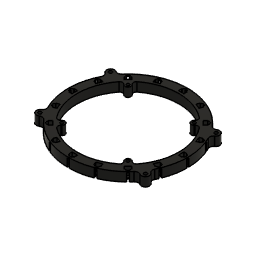
ir_ring_v1 (Autodesk Fusion 360 design; units mm, degrees)
Autodesk Fusion 360 part; units mm, degrees
note: some values were not read from the file. Set by a fixed rule: which sketch regions a step uses.
(part 1 of 2)
sketch "Sketch1" plane through (0, 0, 0) normal (0, 1, 0) x (1, 0, 0)
  circle A0 centre (0, 0) radius 105
  line L0 (0, 0) -> (74.2462, 74.2462) construction
  line L1 (0, 0) -> (105, 0) construction
  line L2 (74.2462, 74.2462) -> (56.5685, 91.9239) construction
  line L3 (56.5685, 91.9239) -> (54.4334, 89.7887) construction
  line L4 (54.4334, 89.7887) -> (43.8268, 79.1821)
  line L5 (43.8268, 79.1821) -> (61.5044, 61.5044)
  line L6 (89.7887, 54.4334) -> (79.1821, 43.8268)
  line L7 (79.1821, 43.8268) -> (61.5044, 61.5044)
  line L8 (-54.4334, 89.7887) -> (-43.8268, 79.1821)
  line L9 (-43.8268, 79.1821) -> (-61.5044, 61.5044)
  line L10 (-79.1821, 43.8268) -> (-61.5044, 61.5044)
  line L11 (-89.7887, 54.4334) -> (-79.1821, 43.8268)
  line L12 (-89.7887, -54.4334) -> (-79.1821, -43.8268)
  line L13 (-79.1821, -43.8268) -> (-61.5044, -61.5044)
  line L14 (-43.8268, -79.1821) -> (-61.5044, -61.5044)
  line L15 (-54.4334, -89.7887) -> (-43.8268, -79.1821)
  line L16 (54.4334, -89.7887) -> (43.8268, -79.1821)
  line L17 (43.8268, -79.1821) -> (61.5044, -61.5044)
  line L18 (79.1821, -43.8268) -> (61.5044, -61.5044)
  line L19 (89.7887, -54.4334) -> (79.1821, -43.8268)
  line L20 (61.5044, 61.5044) -> (58.5876, 58.5876) construction
  line L21 (58.5876, 58.5876) -> (47.3623, 69.8129) construction
  circle A1 centre (47.3623, 69.8129) radius 1.65
  circle A2 centre (69.8129, 47.3623) radius 1.65
  circle A3 centre (-47.3623, 69.8129) radius 1.65
  circle A4 centre (-69.8129, 47.3623) radius 1.65
  circle A5 centre (-69.8129, -47.3623) radius 1.65
  circle A6 centre (-47.3623, -69.8129) radius 1.65
  circle A7 centre (47.3623, -69.8129) radius 1.65
  circle A8 centre (69.8129, -47.3623) radius 1.65
  line L22 (0, 0) -> (0, 105) construction
  line L23 (0, 105) -> (45, 105) construction
  line L24 (45, 105) -> (45, 94.8683) construction
  line L25 (45, 94.8683) -> (0, 94.8683) construction
  line L26 (0, 94.8683) -> (0, 69.8683) construction
  line L27 (0, 69.8683) -> (0, 107.8683) construction
  circle A9 centre (0, 107.8683) radius 38
  line L28 (45, 94.8683) -> (23.4509, 77.9676)
  line L29 (-45, 94.8683) -> (-23.4509, 77.9676)
  circle A10 centre (0, 0) radius 61
  line L30 (0, 0) -> (11.9005, 59.8279) construction
  line L31 (7.9774, 60.6083) -> (6.8068, 54.7236)
  arc A11 (6.8068, 54.7236) -> (14.6531, 53.1628) centre (10.73, 53.9432) ccw
  line L32 (14.6531, 53.1628) -> (15.8237, 59.0475)
  arc A12 (15.8237, 59.0475) -> (7.9774, 60.6083) centre (11.9005, 59.8279) ccw
  line L33 (11.9005, 59.8279) -> (10.73, 53.9432) construction
  circle A13 centre (10.73, 53.9432) radius 1.65
  line L34 (-60.6083, 7.9774) -> (-54.7236, 6.8068)
  line L35 (-53.1628, 14.6531) -> (-59.0475, 15.8237)
  arc A14 (-54.7236, 6.8068) -> (-53.1628, 14.6531) centre (-53.9432, 10.73) ccw
  circle A15 centre (-53.9432, 10.73) radius 1.65
  line L36 (-7.9774, -60.6083) -> (-6.8068, -54.7236)
  line L37 (-14.6531, -53.1628) -> (-15.8237, -59.0475)
  arc A16 (-6.8068, -54.7236) -> (-14.6531, -53.1628) centre (-10.73, -53.9432) ccw
  circle A17 centre (-10.73, -53.9432) radius 1.65
  line L38 (60.6083, -7.9774) -> (54.7236, -6.8068)
  line L39 (53.1628, -14.6531) -> (59.0475, -15.8237)
  arc A18 (54.7236, -6.8068) -> (53.1628, -14.6531) centre (53.9432, -10.73) ccw
  circle A19 centre (53.9432, -10.73) radius 1.65
  dimension "d1" = 210
  dimension "d2" = 45
  dimension "d3" = 25
  dimension "d4" = 15
  dimension "d6" = 360
  dimension "d7" = 4.125
  dimension "d8" = 15.875
  dimension "d9" = 3.3
  dimension "d11" = 360
  dimension "d12" = 45
  dimension "d13" = 25
  dimension "d14" = 38
  dimension "d35" = 122
  dimension "d36" = 11.25
  dimension "d37" = 6
  dimension "d38" = 8
  dimension "d39" = 3.3
  dimension "d41" = 360
  constraint coincident A0.centre L0.start
  constraint horizontal L1
  constraint coincident A0 L0.end
  constraint tangent A0 L2
  constraint coincident A0 L3.end
  constraint perpendicular L2 L3
  constraint perpendicular L2 L4
  constraint coincident L0 L5.end
  constraint perpendicular L0 L5
  constraint symmetric L0 L3.end L6.start
  constraint symmetric L0 L4.end L6.end
  constraint symmetric L0 L5.end L7.end
  constraint perpendicular L7 L20
  constraint perpendicular L20 L21
  constraint coincident L21.end A1.centre
  constraint symmetric L0 A1 A2
  constraint coincident A0 L22.end
  constraint perpendicular L1 L22
  constraint perpendicular L22 L23
  constraint coincident A0 L24.end
  constraint perpendicular L23 L24
  constraint coincident L22 L25.end
  constraint perpendicular L22 L25
  constraint perpendicular L25 L26
  constraint parallel L22 L27
  constraint coincident L27.end A9.centre
  constraint coincident L26.end A9
  constraint coincident A9 L28.end
  constraint tangent A9 L28
  constraint symmetric L22 L24.end L29.start
  constraint symmetric L22 L28.end L29.end
  constraint coincident A10 L30.end
  constraint tangent L31 A11
  constraint tangent A11 L32
  constraint parallel L31 L32
  constraint tangent L32 A12
  constraint tangent L31 A12
  constraint coincident L30 A11.centre
  constraint parallel L30 L33
  constraint coincident L30.end A12.centre
  constraint concentric A11 A13
  measures "d1" diameter of A0
  measures "d2" angle of L0 L1
  measures "d3" distance of L0.end L2.end
  measures "d4" distance of L3.end L4.end
  measures "d7" distance of L5.end L20.end
  measures "d8" distance of L20.end L21.end
  measures "d9" diameter of A1
  measures "d12" distance of L22.end L23.end
  measures "d13" distance of L25.end L26.end
  measures "d14" distance of L26.end L27.end
  measures "d35" diameter of A10
  measures "d36" angle of L22 L30
  measures "d37" distance of L30.end A11.centre
  measures "d38" diameter of A11
  measures "d39" diameter of A13
sketch "Sketch2" plane through (0, 38, 0) normal (0, 1, 0) x (-1, 0, 0)
  circle A0 centre (-69.8129, -47.3623) radius 1.65
  circle A1 centre (-47.3623, -69.8129) radius 1.65
  arc A2 (-50.2791, -72.7297) -> (-44.4455, -66.8961) centre (-47.3623, -69.8129) ccw
  line L0 (-44.4455, -66.8961) -> (-66.8961, -44.4455)
  arc A3 (-66.8961, -44.4455) -> (-72.7297, -50.2791) centre (-69.8129, -47.3623) ccw
  line L1 (-72.7297, -50.2791) -> (-50.2791, -72.7297)
  circle A4 centre (-47.3623, -69.8129) radius 1.65
  circle A5 centre (-69.8129, 47.3623) radius 1.65
  circle A6 centre (-47.3623, 69.8129) radius 1.65
  circle A7 centre (47.3623, 69.8129) radius 1.65
  circle A8 centre (69.8129, 47.3623) radius 1.65
  circle A9 centre (69.8129, -47.3623) radius 1.65
  circle A10 centre (47.3623, -69.8129) radius 1.65
  circle A11 centre (-69.8129, -47.3623) radius 1.65
  line L2 (54.4334, -89.7887) -> (43.8268, -79.1821)
  line L3 (43.8268, -79.1821) -> (79.1821, -43.8268)
  line L4 (79.1821, -43.8268) -> (89.7887, -54.4334)
  arc A12 (89.7887, -54.4334) -> (89.7887, 54.4334) centre (0, 0) ccw
  line L5 (89.7887, 54.4334) -> (79.1821, 43.8268)
  line L6 (79.1821, 43.8268) -> (43.8268, 79.1821)
  line L7 (43.8268, 79.1821) -> (54.4334, 89.7887)
  arc A13 (54.4334, 89.7887) -> (-54.4334, 89.7887) centre (0, 0) ccw
  line L8 (-54.4334, 89.7887) -> (-43.8268, 79.1821)
  line L9 (-43.8268, 79.1821) -> (-79.1821, 43.8268)
  line L10 (-79.1821, 43.8268) -> (-89.7887, 54.4334)
  arc A14 (-89.7887, 54.4334) -> (-89.7887, -54.4334) centre (0, 0) ccw
  line L11 (-89.7887, -54.4334) -> (-79.1821, -43.8268)
  line L12 (-79.1821, -43.8268) -> (-43.8268, -79.1821)
  line L13 (-43.8268, -79.1821) -> (-54.4334, -89.7887)
  arc A15 (-54.4334, -89.7887) -> (-45, -94.8683) centre (0, 0) ccw
  line L14 (-45, -94.8683) -> (-23.4509, -77.9676)
  arc A16 (23.4509, -77.9676) -> (-23.4509, -77.9676) centre (0, -107.8683) ccw
  line L15 (23.4509, -77.9676) -> (45, -94.8683)
  arc A17 (45, -94.8683) -> (54.4334, -89.7887) centre (0, 0) ccw
  line L16 (-79.1821, -43.8268) -> (-82.7176, -40.2912)
  line L17 (-43.8268, -79.1821) -> (-40.2912, -82.7176)
  line L18 (-40.2912, -82.7176) -> (-49.938, -92.3645)
  line L19 (-82.7176, -40.2912) -> (-92.3645, -49.938)
  line L20 (43.8268, -79.1821) -> (40.2912, -82.7176)
  line L21 (40.2912, -82.7176) -> (49.938, -92.3645)
  line L22 (82.7176, -40.2912) -> (92.3645, -49.938)
  line L23 (79.1821, -43.8268) -> (82.7176, -40.2912)
  line L24 (79.1821, 43.8268) -> (82.7176, 40.2912)
  line L25 (82.7176, 40.2912) -> (92.3645, 49.938)
  line L26 (40.2912, 82.7176) -> (49.938, 92.3645)
  line L27 (43.8268, 79.1821) -> (40.2912, 82.7176)
  line L28 (-43.8268, 79.1821) -> (-40.2912, 82.7176)
  line L29 (-40.2912, 82.7176) -> (-49.938, 92.3645)
  line L30 (-82.7176, 40.2912) -> (-92.3645, 49.938)
  line L31 (-79.1821, 43.8268) -> (-82.7176, 40.2912)
  circle A18 centre (-25.9723, -48.5997) radius 1.65
  circle A19 centre (-48.5997, -25.9723) radius 1.65
  circle A20 centre (25.9723, -48.5997) radius 1.65
  circle A21 centre (48.5997, -25.9723) radius 1.65
  circle A22 centre (25.9723, 48.5997) radius 1.65
  circle A23 centre (48.5997, 25.9723) radius 1.65
  circle A24 centre (-25.9723, 48.5997) radius 1.65
  circle A25 centre (-48.5997, 25.9723) radius 1.65
  circle A26 centre (-53.9432, 10.73) radius 1.65
  circle A27 centre (10.73, 53.9432) radius 1.65
  circle A28 centre (53.9432, -10.73) radius 1.65
  circle A29 centre (-10.73, -53.9432) radius 1.65
  arc A30 (-60.4795, 7.9518) -> (-15.798, -58.9188) centre (0, 0) ccw
  line L32 (-60.4795, 7.9518) -> (-54.7236, 6.8068)
  arc A31 (-54.7236, 6.8068) -> (-53.1628, 14.6531) centre (-53.9432, 10.73) ccw
  line L33 (-53.1628, 14.6531) -> (-58.9188, 15.798)
  arc A32 (7.9518, 60.4795) -> (-58.9188, 15.798) centre (0, 0) ccw
  line L34 (7.9518, 60.4795) -> (6.8068, 54.7236)
  arc A33 (6.8068, 54.7236) -> (14.6531, 53.1628) centre (10.73, 53.9432) ccw
  line L35 (14.6531, 53.1628) -> (15.798, 58.9188)
  arc A34 (60.4795, -7.9518) -> (15.798, 58.9188) centre (0, 0) ccw
  line L36 (60.4795, -7.9518) -> (54.7236, -6.8068)
  arc A35 (54.7236, -6.8068) -> (53.1628, -14.6531) centre (53.9432, -10.73) ccw
  line L37 (53.1628, -14.6531) -> (58.9188, -15.798)
  arc A36 (-7.9518, -60.4795) -> (58.9188, -15.798) centre (0, 0) ccw
  line L38 (-7.9518, -60.4795) -> (-6.8068, -54.7236)
  arc A37 (-6.8068, -54.7236) -> (-14.6531, -53.1628) centre (-10.73, -53.9432) ccw
  line L39 (-14.6531, -53.1628) -> (-15.798, -58.9188)
  dimension "d29" = 5
  dimension "d30" = 5
  dimension "d32" = 360
  constraint coincident L11.end L12.start
  constraint perpendicular L11 L16
  constraint coincident L12.end L13.start
  constraint perpendicular L13 L17
  constraint coincident A14 L19.end
  constraint perpendicular L16 L19
  constraint parallel L13 L18
  constraint coincident A15 L18.end
  measures "d29" distance of L11.end L16.end
  measures "d30" distance of L12.end L17.end
sketch "Sketch3" plane through (0, 0, 0) normal (0, -1, 0) x (1, 0, 0)
  circle A0 centre (47.3623, -69.8129) radius 1.65
  circle A1 centre (53.9432, 10.73) radius 1.65
  circle A2 centre (-10.73, 53.9432) radius 1.65
  circle A3 centre (-53.9432, -10.73) radius 1.65
  circle A4 centre (69.8129, -47.3623) radius 1.65
  circle A5 centre (10.73, -53.9432) radius 1.65
  circle A6 centre (69.8129, 47.3623) radius 1.65
  circle A7 centre (47.3623, 69.8129) radius 1.65
  circle A8 centre (-47.3623, 69.8129) radius 1.65
  circle A9 centre (-69.8129, 47.3623) radius 1.65
  circle A10 centre (-69.8129, -47.3623) radius 1.65
  circle A11 centre (-47.3623, -69.8129) radius 1.65
  arc A12 (15.3738, -56.786) -> (17.923, -58.3075) centre (17.3354, -56.3958) ccw
  line L0 (15.3738, -56.786) -> (14.6531, -53.1628)
  arc A13 (14.6531, -53.1628) -> (6.8068, -54.7236) centre (10.73, -53.9432) ccw
  line L1 (6.8068, -54.7236) -> (7.5275, -58.3467)
  arc A14 (5.7546, -60.728) -> (7.5275, -58.3467) centre (5.5659, -58.7369) ccw
  arc A15 (-58.3075, -17.923) -> (5.7546, -60.728) centre (0, 0) ccw
  arc A16 (-56.786, -15.3738) -> (-58.3075, -17.923) centre (-56.3958, -17.3354) ccw
  line L2 (-56.786, -15.3738) -> (-53.1628, -14.6531)
  arc A17 (-53.1628, -14.6531) -> (-54.7236, -6.8068) centre (-53.9432, -10.73) ccw
  line L3 (-54.7236, -6.8068) -> (-58.3467, -7.5275)
  arc A18 (-60.728, -5.7546) -> (-58.3467, -7.5275) centre (-58.7369, -5.5659) ccw
  arc A19 (-17.923, 58.3075) -> (-60.728, -5.7546) centre (0, 0) ccw
  arc A20 (-15.3738, 56.786) -> (-17.923, 58.3075) centre (-17.3354, 56.3958) ccw
  line L4 (-15.3738, 56.786) -> (-14.6531, 53.1628)
  arc A21 (-14.6531, 53.1628) -> (-6.8068, 54.7236) centre (-10.73, 53.9432) ccw
  line L5 (-6.8068, 54.7236) -> (-7.5275, 58.3467)
  arc A22 (-5.7546, 60.728) -> (-7.5275, 58.3467) centre (-5.5659, 58.7369) ccw
  arc A23 (58.3075, 17.923) -> (-5.7546, 60.728) centre (0, 0) ccw
  arc A24 (56.786, 15.3738) -> (58.3075, 17.923) centre (56.3958, 17.3354) ccw
  line L6 (56.786, 15.3738) -> (53.1628, 14.6531)
  arc A25 (53.1628, 14.6531) -> (54.7236, 6.8068) centre (53.9432, 10.73) ccw
  line L7 (54.7236, 6.8068) -> (58.3467, 7.5275)
  arc A26 (60.728, 5.7546) -> (58.3467, 7.5275) centre (58.7369, 5.5659) ccw
  arc A27 (17.923, -58.3075) -> (60.728, 5.7546) centre (0, 0) ccw
  arc A28 (-46.1329, -94.3226) -> (-44.02, -94.0997) centre (-45.2542, -92.526) ccw
  line L8 (-44.02, -94.0997) -> (-23.4509, -77.9676)
  arc A29 (23.4509, -77.9676) -> (-23.4509, -77.9676) centre (0, -107.8683) ccw
  line L9 (23.4509, -77.9676) -> (44.02, -94.0997)
  arc A30 (44.02, -94.0997) -> (46.1329, -94.3226) centre (45.2542, -92.526) ccw
  arc A31 (46.1329, -94.3226) -> (52.1873, -91.1125) centre (0, 0) ccw
  arc A32 (52.1873, -91.1125) -> (52.6075, -87.9628) centre (51.1933, -89.377) ccw
  line L10 (52.6075, -87.9628) -> (45.241, -80.5963)
  arc A33 (45.241, -77.7679) -> (45.241, -80.5963) centre (46.6552, -79.1821) ccw
  line L11 (45.241, -77.7679) -> (77.7679, -45.241)
  arc A34 (80.5963, -45.241) -> (77.7679, -45.241) centre (79.1821, -46.6552) ccw
  line L12 (80.5963, -45.241) -> (87.9628, -52.6075)
  arc A35 (87.9628, -52.6075) -> (91.1125, -52.1873) centre (89.377, -51.1933) ccw
  arc A36 (91.1125, -52.1873) -> (91.1125, 52.1873) centre (0, 0) ccw
  arc A37 (91.1125, 52.1873) -> (87.9628, 52.6075) centre (89.377, 51.1933) ccw
  line L13 (87.9628, 52.6075) -> (80.5963, 45.241)
  arc A38 (77.7679, 45.241) -> (80.5963, 45.241) centre (79.1821, 46.6552) ccw
  line L14 (77.7679, 45.241) -> (45.241, 77.7679)
  arc A39 (45.241, 80.5963) -> (45.241, 77.7679) centre (46.6552, 79.1821) ccw
  line L15 (45.241, 80.5963) -> (52.6075, 87.9628)
  arc A40 (52.6075, 87.9628) -> (52.1873, 91.1125) centre (51.1933, 89.377) ccw
  arc A41 (52.1873, 91.1125) -> (-52.1873, 91.1125) centre (0, 0) ccw
  arc A42 (-52.1873, 91.1125) -> (-52.6075, 87.9628) centre (-51.1933, 89.377) ccw
  line L16 (-52.6075, 87.9628) -> (-45.241, 80.5963)
  arc A43 (-45.241, 77.7679) -> (-45.241, 80.5963) centre (-46.6552, 79.1821) ccw
  line L17 (-45.241, 77.7679) -> (-77.7679, 45.241)
  arc A44 (-80.5963, 45.241) -> (-77.7679, 45.241) centre (-79.1821, 46.6552) ccw
  line L18 (-80.5963, 45.241) -> (-87.9628, 52.6075)
  arc A45 (-87.9628, 52.6075) -> (-91.1125, 52.1873) centre (-89.377, 51.1933) ccw
  arc A46 (-91.1125, 52.1873) -> (-91.1125, -52.1873) centre (0, 0) ccw
  arc A47 (-91.1125, -52.1873) -> (-87.9628, -52.6075) centre (-89.377, -51.1933) ccw
  line L19 (-87.9628, -52.6075) -> (-80.5963, -45.241)
  arc A48 (-77.7679, -45.241) -> (-80.5963, -45.241) centre (-79.1821, -46.6552) ccw
  line L20 (-77.7679, -45.241) -> (-45.241, -77.7679)
  arc A49 (-45.241, -80.5963) -> (-45.241, -77.7679) centre (-46.6552, -79.1821) ccw
  line L21 (-45.241, -80.5963) -> (-52.6075, -87.9628)
  arc A50 (-52.6075, -87.9628) -> (-52.1873, -91.1125) centre (-51.1933, -89.377) ccw
  arc A51 (-52.1873, -91.1125) -> (-46.1329, -94.3226) centre (0, 0) ccw
  circle A52 centre (0, 0) radius 60
  circle A53 centre (0, 0) radius 40
  dimension "d46" = 120
  dimension "d47" = 80
  constraint coincident A15.centre A19.centre
  constraint concentric A52 A53
  measures "d46" diameter of A52
  measures "d47" diameter of A53
sketch "Sketch4" plane through (0, 41, 0) normal (0, 1, 0) x (-1, 0, 0)
  arc A0 (-46.1329, -94.3226) -> (-44.02, -94.0997) centre (-45.2542, -92.526) ccw
  line L0 (-44.02, -94.0997) -> (-23.4509, -77.9676)
  arc A1 (23.4509, -77.9676) -> (-23.4509, -77.9676) centre (0, -107.8683) ccw
  line L1 (23.4509, -77.9676) -> (44.02, -94.0997)
  arc A2 (44.02, -94.0997) -> (46.1329, -94.3226) centre (45.2542, -92.526) ccw
  arc A3 (46.1329, -94.3226) -> (47.5053, -93.6389) centre (0, 0) ccw
  arc A4 (47.5053, -93.6389) -> (48.0147, -90.4411) centre (46.6005, -91.8553) ccw
  line L2 (48.0147, -90.4411) -> (41.7054, -84.1318)
  arc A5 (41.7054, -81.3034) -> (41.7054, -84.1318) centre (43.1196, -82.7176) ccw
  line L3 (41.7054, -81.3034) -> (81.3034, -41.7054)
  arc A6 (84.1318, -41.7054) -> (81.3034, -41.7054) centre (82.7176, -43.1196) ccw
  line L4 (84.1318, -41.7054) -> (90.4411, -48.0147)
  arc A7 (90.4411, -48.0147) -> (93.6389, -47.5053) centre (91.8553, -46.6005) ccw
  arc A8 (93.6389, -47.5053) -> (93.6389, 47.5053) centre (0, 0) ccw
  arc A9 (93.6389, 47.5053) -> (90.4411, 48.0147) centre (91.8553, 46.6005) ccw
  line L5 (90.4411, 48.0147) -> (84.1318, 41.7054)
  arc A10 (81.3034, 41.7054) -> (84.1318, 41.7054) centre (82.7176, 43.1196) ccw
  line L6 (81.3034, 41.7054) -> (41.7054, 81.3034)
  arc A11 (41.7054, 84.1318) -> (41.7054, 81.3034) centre (43.1196, 82.7176) ccw
  line L7 (41.7054, 84.1318) -> (48.0147, 90.4411)
  arc A12 (48.0147, 90.4411) -> (47.5053, 93.6389) centre (46.6005, 91.8553) ccw
  arc A13 (47.5053, 93.6389) -> (-47.5053, 93.6389) centre (0, 0) ccw
  arc A14 (-47.5053, 93.6389) -> (-48.0147, 90.4411) centre (-46.6005, 91.8553) ccw
  line L8 (-48.0147, 90.4411) -> (-41.7054, 84.1318)
  arc A15 (-41.7054, 81.3034) -> (-41.7054, 84.1318) centre (-43.1196, 82.7176) ccw
  line L9 (-41.7054, 81.3034) -> (-81.3034, 41.7054)
  arc A16 (-84.1318, 41.7054) -> (-81.3034, 41.7054) centre (-82.7176, 43.1196) ccw
  line L10 (-84.1318, 41.7054) -> (-90.4411, 48.0147)
  arc A17 (-90.4411, 48.0147) -> (-93.6389, 47.5053) centre (-91.8553, 46.6005) ccw
  arc A18 (-93.6389, 47.5053) -> (-93.6389, -47.5053) centre (0, 0) ccw
  arc A19 (-93.6389, -47.5053) -> (-90.4411, -48.0147) centre (-91.8553, -46.6005) ccw
  line L11 (-90.4411, -48.0147) -> (-84.1318, -41.7054)
  arc A20 (-81.3034, -41.7054) -> (-84.1318, -41.7054) centre (-82.7176, -43.1196) ccw
  line L12 (-81.3034, -41.7054) -> (-41.7054, -81.3034)
  arc A21 (-41.7054, -84.1318) -> (-41.7054, -81.3034) centre (-43.1196, -82.7176) ccw
  line L13 (-41.7054, -84.1318) -> (-48.0147, -90.4411)
  arc A22 (-48.0147, -90.4411) -> (-47.5053, -93.6389) centre (-46.6005, -91.8553) ccw
  arc A23 (-47.5053, -93.6389) -> (-46.1329, -94.3226) centre (0, 0) ccw
  circle A24 centre (-47.3623, -69.8129) radius 1.65
  circle A25 centre (-69.8129, 47.3623) radius 1.65
  circle A26 centre (-47.3623, 69.8129) radius 1.65
  circle A27 centre (47.3623, 69.8129) radius 1.65
  circle A28 centre (69.8129, 47.3623) radius 1.65
  circle A29 centre (69.8129, -47.3623) radius 1.65
  circle A30 centre (47.3623, -69.8129) radius 1.65
  circle A31 centre (-69.8129, -47.3623) radius 1.65
  circle A32 centre (-25.9723, -48.5997) radius 1.65
  circle A33 centre (-48.5997, -25.9723) radius 1.65
  circle A34 centre (25.9723, -48.5997) radius 1.65
  circle A35 centre (48.5997, -25.9723) radius 1.65
  circle A36 centre (25.9723, 48.5997) radius 1.65
  circle A37 centre (48.5997, 25.9723) radius 1.65
  circle A38 centre (-25.9723, 48.5997) radius 1.65
  circle A39 centre (-48.5997, 25.9723) radius 1.65
  line L14 (0, 0) -> (0, -69.8683) construction
  line L15 (0, 0) -> (-10.73, -53.9432) construction
  circle A40 centre (-10.73, -53.9432) radius 1.65
  circle A41 centre (-10.73, -53.9432) radius 2.75
  circle A42 centre (53.9432, -10.73) radius 1.65
  circle A43 centre (53.9432, -10.73) radius 2.75
  circle A44 centre (10.73, 53.9432) radius 1.65
  circle A45 centre (10.73, 53.9432) radius 2.75
  circle A46 centre (-53.9432, 10.73) radius 1.65
  circle A47 centre (-53.9432, 10.73) radius 2.75
  dimension "d50" = 55
  dimension "d51" = 11.25
  dimension "d52" = 3.3
  dimension "d53" = 5.5
  dimension "d55" = 360
  constraint coincident A3.centre A8.centre
  constraint midpoint A1 L14.end
  constraint coincident L15.end A40.centre
  measures "d50" distance of A3.centre L15.end
  measures "d51" angle of L14 L15
  measures "d52" diameter of A40
  measures "d53" diameter of A41
sketch "Sketch5" plane through (0, 61, 0) normal (0, 1, 0) x (-1, 0, 0)
  circle A0 centre (-10.73, -53.9432) radius 1.65
  circle A1 centre (-53.9432, 10.73) radius 1.65
  circle A2 centre (10.73, 53.9432) radius 1.65
  circle A3 centre (53.9432, -10.73) radius 1.65
  circle A4 centre (-10.73, -53.9432) radius 1.65
  circle A5 centre (0, 0) radius 51
  circle A6 centre (0, 0) radius 60
  line L0 (0, 0) -> (0, -55) construction
  line L1 (-2.5, -56.4) -> (2.5, -56.4)
  line L2 (2.5, -56.4) -> (2.5, -53.6)
  line L3 (2.5, -53.6) -> (-2.5, -53.6)
  line L4 (-2.5, -53.6) -> (-2.5, -56.4)
  line L5 (-2.5, -56.4) -> (2.5, -53.6) construction
  line L6 (2.5, -56.4) -> (-2.5, -53.6) construction
  circle A7 centre (0, -56.4) radius 2
  circle A8 centre (0, -56.4) radius 2.2
  line L7 (2.5, -56.4) -> (2.5, -53.6)
  line L8 (2.5, -53.6) -> (-2.5, -53.6)
  line L9 (-2.5, -53.6) -> (-2.5, -56.4)
  line L10 (-2.5, -56.4) -> (2.5, -56.4)
  line L11 (2.7, -56.6) -> (2.7, -53.4)
  line L12 (2.7, -53.4) -> (-2.7, -53.4)
  line L13 (-2.7, -53.4) -> (-2.7, -56.6)
  line L14 (-2.7, -56.6) -> (2.7, -56.6)
  circle A9 centre (21.5833, -52.1068) radius 2.2
  line L15 (17.9408, -50.3684) -> (19.1654, -53.3248)
  line L16 (19.1654, -53.3248) -> (24.1544, -51.2583)
  line L17 (24.1544, -51.2583) -> (22.9298, -48.3019)
  line L18 (22.9298, -48.3019) -> (17.9408, -50.3684)
  circle A10 centre (39.8808, -39.8808) radius 2.2
  line L19 (35.8503, -39.6687) -> (38.1131, -41.9314)
  line L20 (38.1131, -41.9314) -> (41.9314, -38.1131)
  line L21 (41.9314, -38.1131) -> (39.6687, -35.8503)
  line L22 (39.6687, -35.8503) -> (35.8503, -39.6687)
  circle A11 centre (52.1068, -21.5833) radius 2.2
  line L23 (48.3019, -22.9298) -> (51.2583, -24.1544)
  line L24 (51.2583, -24.1544) -> (53.3248, -19.1654)
  line L25 (53.3248, -19.1654) -> (50.3684, -17.9408)
  line L26 (50.3684, -17.9408) -> (48.3019, -22.9298)
  circle A12 centre (56.4, 0) radius 2.2
  line L27 (53.4, -2.7) -> (56.6, -2.7)
  line L28 (56.6, -2.7) -> (56.6, 2.7)
  line L29 (56.6, 2.7) -> (53.4, 2.7)
  line L30 (53.4, 2.7) -> (53.4, -2.7)
  circle A13 centre (52.1068, 21.5833) radius 2.2
  line L31 (50.3684, 17.9408) -> (53.3248, 19.1654)
  line L32 (53.3248, 19.1654) -> (51.2583, 24.1544)
  line L33 (51.2583, 24.1544) -> (48.3019, 22.9298)
  line L34 (48.3019, 22.9298) -> (50.3684, 17.9408)
  circle A14 centre (39.8808, 39.8808) radius 2.2
  line L35 (39.6687, 35.8503) -> (41.9314, 38.1131)
  line L36 (41.9314, 38.1131) -> (38.1131, 41.9314)
  line L37 (38.1131, 41.9314) -> (35.8503, 39.6687)
  line L38 (35.8503, 39.6687) -> (39.6687, 35.8503)
  circle A15 centre (21.5833, 52.1068) radius 2.2
  line L39 (22.9298, 48.3019) -> (24.1544, 51.2583)
  line L40 (24.1544, 51.2583) -> (19.1654, 53.3248)
  line L41 (19.1654, 53.3248) -> (17.9408, 50.3684)
  line L42 (17.9408, 50.3684) -> (22.9298, 48.3019)
  circle A16 centre (0, 56.4) radius 2.2
  line L43 (2.7, 53.4) -> (2.7, 56.6)
  line L44 (2.7, 56.6) -> (-2.7, 56.6)
  line L45 (-2.7, 56.6) -> (-2.7, 53.4)
  line L46 (-2.7, 53.4) -> (2.7, 53.4)
  circle A17 centre (-21.5833, 52.1068) radius 2.2
  line L47 (-17.9408, 50.3684) -> (-19.1654, 53.3248)
  line L48 (-19.1654, 53.3248) -> (-24.1544, 51.2583)
  line L49 (-24.1544, 51.2583) -> (-22.9298, 48.3019)
  line L50 (-22.9298, 48.3019) -> (-17.9408, 50.3684)
  circle A18 centre (-39.8808, 39.8808) radius 2.2
  line L51 (-35.8503, 39.6687) -> (-38.1131, 41.9314)
  line L52 (-38.1131, 41.9314) -> (-41.9314, 38.1131)
  line L53 (-41.9314, 38.1131) -> (-39.6687, 35.8503)
  line L54 (-39.6687, 35.8503) -> (-35.8503, 39.6687)
  circle A19 centre (-52.1068, 21.5833) radius 2.2
  line L55 (-48.3019, 22.9298) -> (-51.2583, 24.1544)
  line L56 (-51.2583, 24.1544) -> (-53.3248, 19.1654)
  line L57 (-53.3248, 19.1654) -> (-50.3684, 17.9408)
  line L58 (-50.3684, 17.9408) -> (-48.3019, 22.9298)
  circle A20 centre (-56.4, 0) radius 2.2
  line L59 (-53.4, 2.7) -> (-56.6, 2.7)
  line L60 (-56.6, 2.7) -> (-56.6, -2.7)
  line L61 (-56.6, -2.7) -> (-53.4, -2.7)
  line L62 (-53.4, -2.7) -> (-53.4, 2.7)
  circle A21 centre (-52.1068, -21.5833) radius 2.2
  line L63 (-50.3684, -17.9408) -> (-53.3248, -19.1654)
  line L64 (-53.3248, -19.1654) -> (-51.2583, -24.1544)
  line L65 (-51.2583, -24.1544) -> (-48.3019, -22.9298)
  line L66 (-48.3019, -22.9298) -> (-50.3684, -17.9408)
  circle A22 centre (-39.8808, -39.8808) radius 2.2
  line L67 (-39.6687, -35.8503) -> (-41.9314, -38.1131)
  line L68 (-41.9314, -38.1131) -> (-38.1131, -41.9314)
  line L69 (-38.1131, -41.9314) -> (-35.8503, -39.6687)
  line L70 (-35.8503, -39.6687) -> (-39.6687, -35.8503)
  circle A23 centre (-21.5833, -52.1068) radius 2.2
  line L71 (-22.9298, -48.3019) -> (-24.1544, -51.2583)
  line L72 (-24.1544, -51.2583) -> (-19.1654, -53.3248)
  line L73 (-19.1654, -53.3248) -> (-17.9408, -50.3684)
  line L74 (-17.9408, -50.3684) -> (-22.9298, -48.3019)
  point P0 (0, -55)
  dimension "d60" = 102
  dimension "d61" = 120
  dimension "d62" = 55
  dimension "d63" = 5
  dimension "d64" = 2.8
  dimension "d65" = 4
  dimension "d66" = 0.2
  dimension "d67" = 0
  dimension "d68" = 0.2
  dimension "d70" = 360
  constraint coincident A5.centre A6.centre
  constraint vertical L0
  constraint horizontal L1
  constraint perpendicular L1 L2
  constraint parallel L1 L3
  constraint parallel L2 L4
  constraint coincident L5 P0
  constraint coincident L6 P0
  constraint coincident P0 L0.end
  constraint midpoint L1 A7.centre
  measures "d60" diameter of A5
  measures "d61" diameter of A6
  measures "d62" distance of A5.centre P0
  measures "d63" distance of L2.end L3.end
  measures "d64" distance of L1.end L2.end
  measures "d65" diameter of A7
  measures "d67" distance of L2
extrude "Extrude6" add sketch "Sketch5" along normal blind 9 makes body 1
sketch "Sketch6" plane through (0, 61, 0) normal (0, -1, 0) x (1, 0, 0)
  circle A0 centre (0, 0) radius 60
  circle A1 centre (0, 0) radius 51
extrude "Extrude7" add sketch "Sketch6" against normal blind 1 bodies 1
ref_plane "WorkPlane1" through (0, 69, 0) normal (0, 1, 0) x (-1, 0, 0)
sketch "Sketch7" plane through (0, 69, 0) normal (0, 1, 0) x (1, 0, 0)
  arc A0 (2.1909, 56.6) -> (-2.1909, 56.6) centre (0, 56.4) ccw
  line L0 (1, 56.4) -> (-1, 56.4)
  line L1 (-1, 56.4) -> (-1, 60.8)
  line L2 (-1, 60.8) -> (1, 60.8)
  line L3 (1, 60.8) -> (1, 56.4)
  line L4 (1, 56.4) -> (-1, 60.8) construction
  line L5 (-1, 56.4) -> (1, 60.8) construction
  line L6 (-22.3433, 56.5546) -> (-20.6595, 52.4895)
  line L7 (-24.191, 55.7892) -> (-22.3433, 56.5546)
  line L8 (-22.5072, 51.7241) -> (-24.191, 55.7892)
  line L9 (-20.6595, 52.4895) -> (-22.5072, 51.7241)
  line L10 (-42.285, 43.6992) -> (-39.1737, 40.5879)
  line L11 (-43.6992, 42.285) -> (-42.285, 43.6992)
  line L12 (-40.5879, 39.1737) -> (-43.6992, 42.285)
  line L13 (-39.1737, 40.5879) -> (-40.5879, 39.1737)
  line L14 (-55.7892, 24.191) -> (-51.7241, 22.5072)
  line L15 (-56.5546, 22.3433) -> (-55.7892, 24.191)
  line L16 (-52.4895, 20.6595) -> (-56.5546, 22.3433)
  line L17 (-51.7241, 22.5072) -> (-52.4895, 20.6595)
  line L18 (-60.8, 1) -> (-56.4, 1)
  line L19 (-60.8, -1) -> (-60.8, 1)
  line L20 (-56.4, -1) -> (-60.8, -1)
  line L21 (-56.4, 1) -> (-56.4, -1)
  line L22 (-56.5546, -22.3433) -> (-52.4895, -20.6595)
  line L23 (-55.7892, -24.191) -> (-56.5546, -22.3433)
  line L24 (-51.7241, -22.5072) -> (-55.7892, -24.191)
  line L25 (-52.4895, -20.6595) -> (-51.7241, -22.5072)
  line L26 (-43.6992, -42.285) -> (-40.5879, -39.1737)
  line L27 (-42.285, -43.6992) -> (-43.6992, -42.285)
  line L28 (-39.1737, -40.5879) -> (-42.285, -43.6992)
  line L29 (-40.5879, -39.1737) -> (-39.1737, -40.5879)
  line L30 (-24.191, -55.7892) -> (-22.5072, -51.7241)
  line L31 (-22.3433, -56.5546) -> (-24.191, -55.7892)
  line L32 (-20.6595, -52.4895) -> (-22.3433, -56.5546)
  line L33 (-22.5072, -51.7241) -> (-20.6595, -52.4895)
  line L34 (-1, -60.8) -> (-1, -56.4)
  line L35 (1, -60.8) -> (-1, -60.8)
  line L36 (1, -56.4) -> (1, -60.8)
  line L37 (-1, -56.4) -> (1, -56.4)
  line L38 (22.3433, -56.5546) -> (20.6595, -52.4895)
  line L39 (24.191, -55.7892) -> (22.3433, -56.5546)
  line L40 (22.5072, -51.7241) -> (24.191, -55.7892)
  line L41 (20.6595, -52.4895) -> (22.5072, -51.7241)
  line L42 (42.285, -43.6992) -> (39.1737, -40.5879)
  line L43 (43.6992, -42.285) -> (42.285, -43.6992)
  line L44 (40.5879, -39.1737) -> (43.6992, -42.285)
  line L45 (39.1737, -40.5879) -> (40.5879, -39.1737)
  line L46 (55.7892, -24.191) -> (51.7241, -22.5072)
  line L47 (56.5546, -22.3433) -> (55.7892, -24.191)
  line L48 (52.4895, -20.6595) -> (56.5546, -22.3433)
  line L49 (51.7241, -22.5072) -> (52.4895, -20.6595)
  line L50 (60.8, -1) -> (56.4, -1)
  line L51 (60.8, 1) -> (60.8, -1)
  line L52 (56.4, 1) -> (60.8, 1)
  line L53 (56.4, -1) -> (56.4, 1)
  line L54 (56.5546, 22.3433) -> (52.4895, 20.6595)
  line L55 (55.7892, 24.191) -> (56.5546, 22.3433)
  line L56 (51.7241, 22.5072) -> (55.7892, 24.191)
  line L57 (52.4895, 20.6595) -> (51.7241, 22.5072)
  line L58 (43.6992, 42.285) -> (40.5879, 39.1737)
  line L59 (42.285, 43.6992) -> (43.6992, 42.285)
  line L60 (39.1737, 40.5879) -> (42.285, 43.6992)
  line L61 (40.5879, 39.1737) -> (39.1737, 40.5879)
  line L62 (24.191, 55.7892) -> (22.5072, 51.7241)
  line L63 (22.3433, 56.5546) -> (24.191, 55.7892)
  line L64 (20.6595, 52.4895) -> (22.3433, 56.5546)
  line L65 (22.5072, 51.7241) -> (20.6595, 52.4895)
  point P0 (0, 58.6)
  dimension "d76" = 2
  dimension "d77" = 4.4
  dimension "d79" = 360
  constraint horizontal L0
  constraint perpendicular L0 L1
  constraint parallel L0 L2
  constraint parallel L1 L3
  constraint coincident L4 P0
  constraint coincident L5 P0
  constraint midpoint A0 P0
  measures "d76" distance of L1.end L2.end
  measures "d77" distance of L0.end L1.end
extrude "Extrude8" cut sketch "Sketch7" against normal blind 8 bodies 1
sketch "Sketch8" plane through (0, 41, 0) normal (0, 1, 0) x (-1, 0, 0)
  circle A0 centre (53.9432, -10.73) radius 1.65
  circle A1 centre (-53.9432, 10.73) radius 1.65
  circle A2 centre (-10.73, -53.9432) radius 1.65
  circle A3 centre (10.73, 53.9432) radius 1.65
  arc A4 (-46.1329, -94.3226) -> (-44.02, -94.0997) centre (-45.2542, -92.526) ccw
  line L0 (-44.02, -94.0997) -> (-23.4509, -77.9676)
  arc A5 (23.4509, -77.9676) -> (-23.4509, -77.9676) centre (0, -107.8683) ccw
  line L1 (23.4509, -77.9676) -> (44.02, -94.0997)
  arc A6 (44.02, -94.0997) -> (46.1329, -94.3226) centre (45.2542, -92.526) ccw
  arc A7 (46.1329, -94.3226) -> (47.5053, -93.6389) centre (0, 0) ccw
  arc A8 (47.5053, -93.6389) -> (48.0147, -90.4411) centre (46.6005, -91.8553) ccw
  line L2 (48.0147, -90.4411) -> (41.7054, -84.1318)
  arc A9 (41.7054, -81.3034) -> (41.7054, -84.1318) centre (43.1196, -82.7176) ccw
  line L3 (41.7054, -81.3034) -> (81.3034, -41.7054)
  arc A10 (84.1318, -41.7054) -> (81.3034, -41.7054) centre (82.7176, -43.1196) ccw
  line L4 (84.1318, -41.7054) -> (90.4411, -48.0147)
  arc A11 (90.4411, -48.0147) -> (93.6389, -47.5053) centre (91.8553, -46.6005) ccw
  arc A12 (93.6389, -47.5053) -> (93.6389, 47.5053) centre (0, 0) ccw
  arc A13 (93.6389, 47.5053) -> (90.4411, 48.0147) centre (91.8553, 46.6005) ccw
  line L5 (90.4411, 48.0147) -> (84.1318, 41.7054)
  arc A14 (81.3034, 41.7054) -> (84.1318, 41.7054) centre (82.7176, 43.1196) ccw
  line L6 (81.3034, 41.7054) -> (41.7054, 81.3034)
  arc A15 (41.7054, 84.1318) -> (41.7054, 81.3034) centre (43.1196, 82.7176) ccw
  line L7 (41.7054, 84.1318) -> (48.0147, 90.4411)
  arc A16 (48.0147, 90.4411) -> (47.5053, 93.6389) centre (46.6005, 91.8553) ccw
  arc A17 (47.5053, 93.6389) -> (-47.5053, 93.6389) centre (0, 0) ccw
  arc A18 (-47.5053, 93.6389) -> (-48.0147, 90.4411) centre (-46.6005, 91.8553) ccw
  line L8 (-48.0147, 90.4411) -> (-41.7054, 84.1318)
  arc A19 (-41.7054, 81.3034) -> (-41.7054, 84.1318) centre (-43.1196, 82.7176) ccw
  line L9 (-41.7054, 81.3034) -> (-81.3034, 41.7054)
  arc A20 (-84.1318, 41.7054) -> (-81.3034, 41.7054) centre (-82.7176, 43.1196) ccw
  line L10 (-84.1318, 41.7054) -> (-90.4411, 48.0147)
  arc A21 (-90.4411, 48.0147) -> (-93.6389, 47.5053) centre (-91.8553, 46.6005) ccw
  arc A22 (-93.6389, 47.5053) -> (-93.6389, -47.5053) centre (0, 0) ccw
  arc A23 (-93.6389, -47.5053) -> (-90.4411, -48.0147) centre (-91.8553, -46.6005) ccw
  line L11 (-90.4411, -48.0147) -> (-84.1318, -41.7054)
  arc A24 (-81.3034, -41.7054) -> (-84.1318, -41.7054) centre (-82.7176, -43.1196) ccw
  line L12 (-81.3034, -41.7054) -> (-41.7054, -81.3034)
  arc A25 (-41.7054, -84.1318) -> (-41.7054, -81.3034) centre (-43.1196, -82.7176) ccw
  line L13 (-41.7054, -84.1318) -> (-48.0147, -90.4411)
  arc A26 (-48.0147, -90.4411) -> (-47.5053, -93.6389) centre (-46.6005, -91.8553) ccw
  arc A27 (-47.5053, -93.6389) -> (-46.1329, -94.3226) centre (0, 0) ccw
  circle A28 centre (-47.3623, -69.8129) radius 1.65
  circle A29 centre (-69.8129, 47.3623) radius 1.65
  circle A30 centre (-47.3623, 69.8129) radius 1.65
  circle A31 centre (47.3623, 69.8129) radius 1.65
  circle A32 centre (69.8129, 47.3623) radius 1.65
  circle A33 centre (69.8129, -47.3623) radius 1.65
  circle A34 centre (47.3623, -69.8129) radius 1.65
  circle A35 centre (-69.8129, -47.3623) radius 1.65
  circle A36 centre (-25.9723, -48.5997) radius 1.65
  circle A37 centre (-48.5997, -25.9723) radius 1.65
  circle A38 centre (25.9723, -48.5997) radius 1.65
  circle A39 centre (48.5997, -25.9723) radius 1.65
  circle A40 centre (25.9723, 48.5997) radius 1.65
  circle A41 centre (48.5997, 25.9723) radius 1.65
  circle A42 centre (-25.9723, 48.5997) radius 1.65
  circle A43 centre (-48.5997, 25.9723) radius 1.65
  line L14 (0, 0) -> (97, 0) construction
  line L15 (0, 0) -> (0, 97) construction
  line L16 (0, 0) -> (-97, 0) construction
  line L17 (0, 0) -> (0, -75) construction
  line L18 (0, -75) -> (35, -75) construction
  line L19 (0, -75) -> (-35, -75) construction
  circle A44 centre (35, -75) radius 1.65
  circle A45 centre (35, -75) radius 2.75
  circle A46 centre (-35, -75) radius 1.65
  circle A47 centre (-35, -75) radius 2.75
  circle A48 centre (97, 0) radius 1.65
  circle A49 centre (97, 0) radius 2.75
  circle A50 centre (-97, 0) radius 1.65
  circle A51 centre (-97, 0) radius 2.75
  circle A52 centre (0, 97) radius 1.65
  circle A53 centre (0, 97) radius 2.75
  dimension "d82" = 97
  dimension "d83" = 97
  dimension "d84" = 97
  dimension "d85" = 75
  dimension "d86" = 35
  dimension "d87" = 35
  dimension "d88" = 3.3
  dimension "d89" = 5.5
  dimension "d90" = 3.3
  dimension "d91" = 5.5
  dimension "d92" = 3.3
  dimension "d93" = 5.5
  dimension "d94" = 3.3
  dimension "d95" = 5.5
  dimension "d96" = 3.3
  dimension "d97" = 5.5
  constraint coincident A7.centre A12.centre
  constraint horizontal L14
  constraint perpendicular L14 L15
  constraint perpendicular L15 L16
  constraint perpendicular L17 L18
  constraint perpendicular L17 L19
  constraint coincident L18.end A44.centre
  constraint coincident L19.end A46.centre
  constraint coincident L14.end A48.centre
  constraint concentric A48 A49
  constraint coincident L16.end A50.centre
  constraint coincident L15.end A52.centre
  constraint concentric A52 A53
  measures "d82" distance of A7.centre L14.end
  measures "d83" distance of A7.centre L15.end
  measures "d84" distance of A7.centre L16.end
  measures "d85" distance of A7.centre L17.end
  measures "d86" distance of L17.end L18.end
  measures "d87" distance of L17.end L19.end
  measures "d88" diameter of A44
  measures "d89" diameter of A45
  measures "d90" diameter of A46
  measures "d91" diameter of A47
  measures "d92" diameter of A48
  measures "d93" diameter of A49
  measures "d94" diameter of A50
  measures "d95" diameter of A51
  measures "d96" diameter of A52
  measures "d97" diameter of A53
sketch "Sketch9" plane through (0, 141, 0) normal (0, 1, 0) x (-1, 0, 0)
  circle A0 centre (35, -75) radius 1.65
  circle A1 centre (0, 0) radius 105
  circle A2 centre (0, 0) radius 92.5
  circle A3 centre (-35, -75) radius 1.65
  circle A4 centre (35, -75) radius 1.65
  circle A5 centre (97, 0) radius 1.65
  circle A6 centre (-97, 0) radius 1.65
  circle A7 centre (0, 97) radius 1.65
  line L0 (35, -75) -> (35, -83) construction
  line L1 (35, -75) -> (35, -67) construction
  line L2 (35, -83) -> (-40.832, -83)
  line L3 (35, -83) -> (40.832, -83)
  line L4 (35, -67) -> (-63.775, -67)
  line L5 (35, -67) -> (63.775, -67)
  line L6 (40.832, -83) -> (64.3117, -83)
  line L7 (63.775, -67) -> (80.8455, -67)
  line L8 (-40.832, -83) -> (-64.3117, -83)
  line L9 (-63.775, -67) -> (-80, -67)
  dimension "d102" = 210
  dimension "d103" = 185
  dimension "d104" = 8
  dimension "d105" = 8
  constraint coincident A1.centre A2.centre
  constraint coincident A0.centre A4.centre
  constraint vertical L0
  constraint parallel L0 L1
  constraint coincident A2 L2.end
  constraint perpendicular L0 L2
  constraint coincident A2 L3.end
  constraint perpendicular L0 L3
  constraint coincident A2 L4.end
  constraint perpendicular L1 L4
  constraint coincident A2 L5.end
  constraint perpendicular L1 L5
  constraint coincident A1 L6.end
  constraint parallel L3 L6
  constraint coincident A1 L7.end
  constraint parallel L5 L7
  constraint coincident A1 L8.end
  constraint parallel L2 L8
  constraint parallel L4 L9
  measures "d102" diameter of A1
  measures "d103" diameter of A2
  measures "d104" distance of A0.centre L0.end
  measures "d105" distance of A0.centre L1.end
extrude "Extrude13" add 4 faces at (-11.2153, 62, 53.5691) (53.4444, 62, 11.4139) (-54.4419, 62, -10.046) (11.1551, 62, -53.5132) along direction (0, 1, 0) blind 8 on bodies 1 bodies 1
sketch "Sketch11" plane through (0, 70, 0) normal (0, 1, 0) x (-1, 0, 0)
  line L0 (-22.9298, -48.3019) -> (-17.9408, -50.3684)
  line L1 (-17.9408, -50.3684) -> (-19.1654, -53.3248)
  line L2 (-19.1654, -53.3248) -> (-19.6358, -53.13)
  arc A0 (-23.684, -51.4532) -> (-19.6358, -53.13) centre (-21.5833, -52.1068) ccw
  line L3 (-23.684, -51.4532) -> (-24.1544, -51.2583)
  line L4 (-24.1544, -51.2583) -> (-22.9298, -48.3019)
  line L5 (22.9298, 48.3019) -> (17.9408, 50.3684)
  line L6 (17.9408, 50.3684) -> (19.1654, 53.3248)
  line L7 (19.1654, 53.3248) -> (19.6358, 53.13)
  arc A1 (23.684, 51.4532) -> (19.6358, 53.13) centre (21.5833, 52.1068) ccw
  line L8 (23.684, 51.4532) -> (24.1544, 51.2583)
  line L9 (24.1544, 51.2583) -> (22.9298, 48.3019)
  line L10 (-17.9408, 50.3684) -> (-22.9298, 48.3019)
  line L11 (-22.9298, 48.3019) -> (-24.1544, 51.2583)
  line L12 (-24.1544, 51.2583) -> (-23.684, 51.4532)
  arc A2 (-19.6358, 53.13) -> (-23.684, 51.4532) centre (-21.5833, 52.1068) ccw
  line L13 (-19.6358, 53.13) -> (-19.1654, 53.3248)
  line L14 (-19.1654, 53.3248) -> (-17.9408, 50.3684)
  line L15 (-48.3019, 22.9298) -> (-50.3684, 17.9408)
  line L16 (-50.3684, 17.9408) -> (-53.3248, 19.1654)
  line L17 (-53.3248, 19.1654) -> (-53.13, 19.6358)
  arc A3 (-51.4532, 23.684) -> (-53.13, 19.6358) centre (-52.1068, 21.5833) ccw
  line L18 (-51.4532, 23.684) -> (-51.2583, 24.1544)
  line L19 (-51.2583, 24.1544) -> (-48.3019, 22.9298)
  line L20 (48.3019, -22.9298) -> (50.3684, -17.9408)
  line L21 (50.3684, -17.9408) -> (53.3248, -19.1654)
  line L22 (53.3248, -19.1654) -> (53.13, -19.6358)
  arc A4 (51.4532, -23.684) -> (53.13, -19.6358) centre (52.1068, -21.5833) ccw
  line L23 (51.4532, -23.684) -> (51.2583, -24.1544)
  line L24 (51.2583, -24.1544) -> (48.3019, -22.9298)
  line L25 (50.3684, 17.9408) -> (48.3019, 22.9298)
  line L26 (48.3019, 22.9298) -> (51.2583, 24.1544)
  line L27 (51.2583, 24.1544) -> (51.4532, 23.684)
  arc A5 (53.13, 19.6358) -> (51.4532, 23.684) centre (52.1068, 21.5833) ccw
  line L28 (53.13, 19.6358) -> (53.3248, 19.1654)
  line L29 (53.3248, 19.1654) -> (50.3684, 17.9408)
  line L30 (-2.1909, -56.6) -> (-2.7, -56.6)
  line L31 (-2.7, -56.6) -> (-2.7, -53.4)
  line L32 (-2.7, -53.4) -> (2.7, -53.4)
  line L33 (2.7, -53.4) -> (2.7, -56.6)
  line L34 (2.7, -56.6) -> (2.1909, -56.6)
  arc A6 (-2.1909, -56.6) -> (2.1909, -56.6) centre (0, -56.4) ccw
  line L35 (39.6687, 35.8503) -> (35.8503, 39.6687)
  line L36 (35.8503, 39.6687) -> (38.1131, 41.9314)
  line L37 (38.1131, 41.9314) -> (38.4731, 41.5714)
  arc A7 (41.5714, 38.4731) -> (38.4731, 41.5714) centre (39.8808, 39.8808) ccw
  line L38 (41.5714, 38.4731) -> (41.9314, 38.1131)
  line L39 (41.9314, 38.1131) -> (39.6687, 35.8503)
  line L40 (17.9408, -50.3684) -> (22.9298, -48.3019)
  line L41 (22.9298, -48.3019) -> (24.1544, -51.2583)
  line L42 (24.1544, -51.2583) -> (23.684, -51.4532)
  arc A8 (19.6358, -53.13) -> (23.684, -51.4532) centre (21.5833, -52.1068) ccw
  line L43 (19.6358, -53.13) -> (19.1654, -53.3248)
  line L44 (19.1654, -53.3248) -> (17.9408, -50.3684)
  line L45 (2.7, 53.4) -> (-2.7, 53.4)
  line L46 (-2.7, 53.4) -> (-2.7, 56.6)
  line L47 (-2.7, 56.6) -> (-2.1909, 56.6)
  arc A9 (2.1909, 56.6) -> (-2.1909, 56.6) centre (0, 56.4) ccw
  line L48 (2.1909, 56.6) -> (2.7, 56.6)
  line L49 (2.7, 56.6) -> (2.7, 53.4)
  line L50 (-35.8503, 39.6687) -> (-39.6687, 35.8503)
  line L51 (-39.6687, 35.8503) -> (-41.9314, 38.1131)
  line L52 (-41.9314, 38.1131) -> (-41.5714, 38.4731)
  arc A10 (-38.4731, 41.5714) -> (-41.5714, 38.4731) centre (-39.8808, 39.8808) ccw
  line L53 (-38.4731, 41.5714) -> (-38.1131, 41.9314)
  line L54 (-38.1131, 41.9314) -> (-35.8503, 39.6687)
  line L55 (-50.3684, -17.9408) -> (-48.3019, -22.9298)
  line L56 (-48.3019, -22.9298) -> (-51.2583, -24.1544)
  line L57 (-51.2583, -24.1544) -> (-51.4532, -23.684)
  arc A11 (-53.13, -19.6358) -> (-51.4532, -23.684) centre (-52.1068, -21.5833) ccw
  line L58 (-53.13, -19.6358) -> (-53.3248, -19.1654)
  line L59 (-53.3248, -19.1654) -> (-50.3684, -17.9408)
  line L60 (35.8503, -39.6687) -> (39.6687, -35.8503)
  line L61 (39.6687, -35.8503) -> (41.9314, -38.1131)
  line L62 (41.9314, -38.1131) -> (41.5714, -38.4731)
  arc A12 (38.4731, -41.5714) -> (41.5714, -38.4731) centre (39.8808, -39.8808) ccw
  line L63 (38.4731, -41.5714) -> (38.1131, -41.9314)
  line L64 (38.1131, -41.9314) -> (35.8503, -39.6687)
  line L65 (53.4, -2.7) -> (53.4, 2.7)
  line L66 (53.4, 2.7) -> (56.6, 2.7)
  line L67 (56.6, 2.7) -> (56.6, 2.1909)
  arc A13 (56.6, -2.1909) -> (56.6, 2.1909) centre (56.4, 0) ccw
  line L68 (56.6, -2.1909) -> (56.6, -2.7)
  line L69 (56.6, -2.7) -> (53.4, -2.7)
  circle A14 centre (0, 0) radius 51
  line L70 (-53.4, 2.7) -> (-53.4, -2.7)
  line L71 (-53.4, -2.7) -> (-56.6, -2.7)
  line L72 (-56.6, -2.7) -> (-56.6, -2.1909)
  arc A15 (-56.6, 2.1909) -> (-56.6, -2.1909) centre (-56.4, 0) ccw
  line L73 (-56.6, 2.1909) -> (-56.6, 2.7)
  line L74 (-56.6, 2.7) -> (-53.4, 2.7)
  line L75 (-39.6687, -35.8503) -> (-35.8503, -39.6687)
  line L76 (-35.8503, -39.6687) -> (-38.1131, -41.9314)
  line L77 (-38.1131, -41.9314) -> (-38.4731, -41.5714)
  arc A16 (-41.5714, -38.4731) -> (-38.4731, -41.5714) centre (-39.8808, -39.8808) ccw
  line L78 (-41.5714, -38.4731) -> (-41.9314, -38.1131)
  line L79 (-41.9314, -38.1131) -> (-39.6687, -35.8503)
  circle A17 centre (0, 0) radius 60
  line L80 (62, 12.5) -> (-62, 12.5)
  line L81 (-62, 12.5) -> (-62, -12.5)
  line L82 (-62, -12.5) -> (62, -12.5)
  line L83 (62, -12.5) -> (62, 12.5)
  line L84 (62, 12.5) -> (-62, -12.5) construction
  line L85 (-62, 12.5) -> (62, -12.5) construction
  circle A18 centre (-62, -12.5) radius 1.5
  circle A19 centre (-62, 12.5) radius 1.5
  circle A20 centre (62, 12.5) radius 1.5
  circle A21 centre (62, -12.5) radius 1.5
  line L86 (62, 12.5) -> (49.994, 10.0794)
  line L87 (57.1874, 11.5297) -> (56.5945, 14.4705)
  line L88 (57.1874, 11.5297) -> (57.7803, 8.5889)
  line L89 (57.7803, 8.5889) -> (65.6225, 10.17)
  line L90 (65.6225, 10.17) -> (64.4367, 16.0516)
  line L91 (56.5945, 14.4705) -> (64.4367, 16.0516)
  line L92 (0, 0) -> (22, 0) construction
  line L93 (0, 0) -> (0, -7) construction
  circle A22 centre (62, -12.5) radius 1.5
  line L94 (65.6225, -10.17) -> (64.4367, -16.0516)
  line L95 (57.7803, -8.5889) -> (65.6225, -10.17)
  line L96 (57.1874, -11.5297) -> (57.7803, -8.5889)
  line L97 (56.5945, -14.4705) -> (64.4367, -16.0516)
  line L98 (57.1874, -11.5297) -> (56.5945, -14.4705)
  circle A23 centre (-62, -12.5) radius 1.5
  line L99 (-57.7803, -8.5889) -> (-65.6225, -10.17)
  line L100 (-57.1874, -11.5297) -> (-57.7803, -8.5889)
  line L101 (-57.1874, -11.5297) -> (-56.5945, -14.4705)
  line L102 (-56.5945, -14.4705) -> (-64.4367, -16.0516)
  line L103 (-65.6225, -10.17) -> (-64.4367, -16.0516)
  line L104 (-57.7803, 8.5889) -> (-65.6225, 10.17)
  line L105 (-57.1874, 11.5297) -> (-57.7803, 8.5889)
  line L106 (-57.1874, 11.5297) -> (-56.5945, 14.4705)
  line L107 (-56.5945, 14.4705) -> (-64.4367, 16.0516)
  circle A24 centre (-62, 12.5) radius 1.5
  line L108 (-65.6225, 10.17) -> (-64.4367, 16.0516)
  point P0 (62, -12.5)
  dimension "d117" = 25
  dimension "d118" = 3
  dimension "d119" = 3
  dimension "d120" = 3
  dimension "d121" = 3
  dimension "d123" = 3
  dimension "d124" = 3
  dimension "d125" = 8
  dimension "d126" = 6
  constraint horizontal L80
  constraint perpendicular L80 L81
  constraint parallel L80 L82
  constraint parallel L81 L83
  constraint coincident L84 A14.centre
  constraint coincident L85 A14.centre
  constraint coincident A14.centre A17.centre
  constraint coincident L81.end L82.start
  constraint coincident L80.end L81.start
  constraint coincident L80.start L83.end
  constraint coincident P0 L82.end
  constraint coincident A14 L86.end
  constraint coincident L84 L86.end
  constraint coincident L86 L87.start
  constraint perpendicular L86 L87
  constraint perpendicular L86 L88
  constraint perpendicular L88 L89
  constraint perpendicular L89 L90
  constraint horizontal L92
  constraint perpendicular L92 L93
  constraint symmetric L80.start L92 P0
  constraint symmetric A20 L92 A22
  constraint symmetric L87.start L92 L96.start
  constraint symmetric L87.end L92 L97.start
  constraint symmetric L88.end L92 L95.start
  constraint symmetric L89.end L92 L94.start
  constraint symmetric L90.end L92 L94.end
  constraint symmetric A20 L93 A24
  constraint symmetric L87.start L93 L105.start
  constraint symmetric L87.end L93 L106.end
  constraint symmetric L88.end L93 L104.start
  constraint symmetric L89.end L93 L104.end
  constraint symmetric L90.end L93 L107.end
  constraint symmetric L93 L94.start L99.end
  constraint symmetric L93 L94.end L102.end
  constraint symmetric L93 L96.start L100.start
  constraint symmetric L93 L97.start L101.end
  constraint symmetric L93 L95.start L99.start
  constraint symmetric L93 A22 A23
  measures "d117" distance of L80.end L81.end
  measures "d118" diameter of A18
  measures "d119" diameter of A19
  measures "d120" diameter of A20
  measures "d121" diameter of A21
  measures "d123" distance of L87.start L87.end
  measures "d124" distance of L87.start L88.end
  measures "d125" distance of L88.end L89.end
  measures "d126" distance of L89.end L90.end